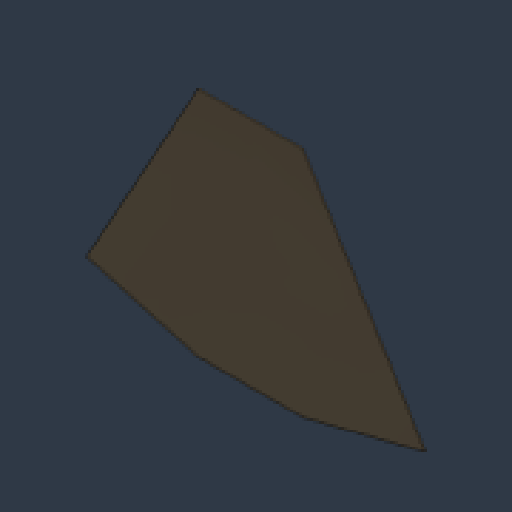
# Autodesk Inventor part: hopper_back_plate
Saved by Autodesk Inventor 2024.3 (Build 283343000, 343)
## iProperties
Created: 2025-03-05
Part Number: hopper_back_plate
Material: Polycarbonate, Smoke
Document SubType Name: Sheet Metal
Designer: Marcus Tannini
Density: 1.2 g/cm^3
Sheet Metal Rule: Default
Appearance: Polycarbonate - Smoked
Mass: 482.78 g
Surface Area: 2692.42 cm^2
Volume: 402.316 cm^3
Author: Marcus Tannini
Autodesk Inventor part; units mm, degrees
ref_plane "YZ Plane" through (0, 0, 0) normal (1, 0, 0) x (0, 1, 0)
ref_plane "XZ Plane" through (0, 0, 0) normal (0, 1, 0) x (-1, 0, 0)
ref_plane "XY Plane" through (0, 0, 0) normal (0, 0, 1) x (1, 0, 0)
sketch "Sketch1" plane through (0, 0, 0) normal (0, 0, 1) x (1, 0, 0)
  line L0 (381.5852, -185.7682) -> (94.217, 105.9508)
  line L1 (94.217, 105.9508) -> (-70.883, 105.9508)
  line L2 (-70.883, 105.9508) -> (-358.2512, -185.7682)
  line L3 (1105.6551, 353.06) -> (-810.8916, 353.06) construction
  line L4 (381.5852, -185.7682) -> (-358.2512, -185.7682)
  dimension "d4" = 165.1
  dimension "d7" = 291.719
  measures "d4" distance of L0.end L1.end
  measures "d7" distance between parallel lines of L4 L1
extrude "Plate1" add sketch "Sketch1" along normal blind 3.048
equation "\"d2\" = Thickness"
equation "\"BendRadius\" = Thickness"
equation "\"BendReliefWidth\" = Thickness"
equation "\"BendReliefDepth\" = 0.5 * Thickness"
equation "\"CornerReliefSize\" = 4 * Thickness"
equation "\"MinimumRemnant\" = 2 * Thickness"
equation "\"TransitionRadius\" = BendRadius"
equation "\"JacobiRadiusSize\" = BendRadius"
equation "\"GapSize\" = Thickness"
equation "\"Thickness\" = 3.048"
body "Solid1"
